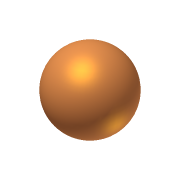
# Autodesk Inventor part: Ball
Saved by Autodesk Inventor 2011 (Build 150239000, 239)
## iProperties
Created: 2011-04-09
Part Number: Ball
Document SubType Name: Modeling
Designer: Milton
Density: 1 g/cm^3
Author: Milton
Autodesk Inventor part; units mm, degrees
ref_plane "YZ Plane" through (0, 0, 0) normal (1, 0, 0) x (0, 1, 0)
ref_plane "XZ Plane" through (0, 0, 0) normal (0, 1, 0) x (-1, 0, 0)
ref_plane "XY Plane" through (0, 0, 0) normal (0, 0, 1) x (1, 0, 0)
sketch "Sketch1" plane through (0, 0, 0) normal (0, 0, 1) x (1, 0, 0)
  circle A0 centre (0, 0) radius 50
  line L0 (0, 50) -> (0, -50)
  dimension "d0" = 100
  constraints: 2 end point, 2 point on circle, 1 centre point, 1 coincident, 1 vertical
  measures "d0" diameter of A0
revolve "Revolution1" add sketch "Sketch1" angle 360 about axis through (0, 50, 0) along (0, -1, 0) picked at (-20.2359, 10.5282) contours L0 A0
body "Solid1"
